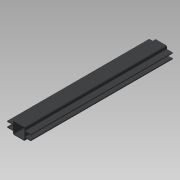
# Autodesk Inventor part: 9035
Saved by Autodesk Inventor 2013 (Build 170138000, 138)
## iProperties
Company: 80/20 Inc.
Created: 2014-04-23
Part Number: 9035
Material: Generic
Document SubType Name: Modeling
Density: 1 g/cm^3
Vendor: 80/20 Inc.
Engineer: Ross Bowman
Designer: Ross Bowman
Catalog Web Link: 8020.net
Material: 6105-T5 Aluminum
Author: Ross Bowman
Keywords: 80/20 , 8020 , T-Slot , Extrusion
Autodesk Inventor part; units mm, degrees
ref_plane "YZ Plane" through (0, 0, 0) normal (1, 0, 0) x (0, 1, 0)
ref_plane "XZ Plane" through (0, 0, 0) normal (0, 1, 0) x (-1, 0, 0)
ref_plane "XY Plane" through (0, 0, 0) normal (0, 0, 1) x (1, 0, 0)
sketch "Sketch1" plane through (0, 0, 0) normal (0, 0, 1) x (1, 0, 0)
  line L0 (-9.652, -11.176) -> (9.652, -11.176)
  arc A0 (-11.176, -9.652) -> (-9.652, -11.176) centre (-9.652, -9.652) ccw
  line L1 (-11.176, 9.652) -> (-11.176, -9.652)
  arc A1 (-9.652, 11.176) -> (-11.176, 9.652) centre (-9.652, 9.652) ccw
  line L2 (9.652, 11.176) -> (-9.652, 11.176)
  arc A2 (11.176, 9.652) -> (9.652, 11.176) centre (9.652, 9.652) ccw
  line L3 (11.176, -9.652) -> (11.176, 9.652)
  arc A3 (9.652, -11.176) -> (11.176, -9.652) centre (9.652, -9.652) ccw
  arc A4 (12.7, 6.731) -> (13.081, 6.35) centre (13.081, 6.731) ccw
  line L4 (12.7, 6.731) -> (12.7, 10.5918)
  arc A5 (12.7, 10.5918) -> (10.5918, 12.7) centre (10.5918, 10.5918) ccw
  line L5 (10.5918, 12.7) -> (-10.5918, 12.7)
  arc A6 (-10.5918, 12.7) -> (-12.7, 10.5918) centre (-10.5918, 10.5918) ccw
  line L6 (-12.7, 10.5918) -> (-12.7, 6.731)
  arc A7 (-13.081, 6.35) -> (-12.7, 6.731) centre (-13.081, 6.731) ccw
  line L7 (-13.081, 6.35) -> (-25.019, 6.35)
  arc A8 (-25.019, 6.35) -> (-25.4, 5.969) centre (-25.019, 5.969) ccw
  line L8 (-25.4, 5.969) -> (-25.4, 4.826)
  arc A9 (-25.4, 4.826) -> (-24.638, 4.064) centre (-24.638, 4.826) ccw
  line L9 (-24.638, 4.064) -> (-23.0632, 4.064)
  arc A10 (-23.0632, 4.064) -> (-22.6822, 4.445) centre (-23.0632, 4.445) ccw
  arc A11 (-22.3012, 4.826) -> (-22.6822, 4.445) centre (-22.3012, 4.445) ccw
  line L10 (-22.3012, 4.826) -> (-13.081, 4.826)
  arc A12 (-12.7, 4.445) -> (-13.081, 4.826) centre (-13.081, 4.445) ccw
  line L11 (-12.7, 4.445) -> (-12.7, -4.445)
  arc A13 (-13.081, -4.826) -> (-12.7, -4.445) centre (-13.081, -4.445) ccw
  line L12 (-13.081, -4.826) -> (-22.3012, -4.826)
  arc A14 (-22.6822, -4.445) -> (-22.3012, -4.826) centre (-22.3012, -4.445) ccw
  arc A15 (-22.6822, -4.445) -> (-23.0632, -4.064) centre (-23.0632, -4.445) ccw
  line L13 (-23.0632, -4.064) -> (-24.638, -4.064)
  arc A16 (-24.638, -4.064) -> (-25.4, -4.826) centre (-24.638, -4.826) ccw
  line L14 (-25.4, -4.826) -> (-25.4, -5.969)
  arc A17 (-25.4, -5.969) -> (-25.019, -6.35) centre (-25.019, -5.969) ccw
  line L15 (-25.019, -6.35) -> (-13.081, -6.35)
  arc A18 (-12.7, -6.731) -> (-13.081, -6.35) centre (-13.081, -6.731) ccw
  line L16 (-12.7, -6.731) -> (-12.7, -10.5918)
  arc A19 (-12.7, -10.5918) -> (-10.5918, -12.7) centre (-10.5918, -10.5918) ccw
  line L17 (-10.5918, -12.7) -> (10.5918, -12.7)
  arc A20 (10.5918, -12.7) -> (12.7, -10.5918) centre (10.5918, -10.5918) ccw
  line L18 (12.7, -10.5918) -> (12.7, -6.731)
  arc A21 (13.081, -6.35) -> (12.7, -6.731) centre (13.081, -6.731) ccw
  line L19 (13.081, -6.35) -> (25.019, -6.35)
  arc A22 (25.019, -6.35) -> (25.4, -5.969) centre (25.019, -5.969) ccw
  line L20 (25.4, -5.969) -> (25.4, -4.826)
  arc A23 (25.4, -4.826) -> (24.638, -4.064) centre (24.638, -4.826) ccw
  line L21 (24.638, -4.064) -> (23.0632, -4.064)
  arc A24 (23.0632, -4.064) -> (22.6822, -4.445) centre (23.0632, -4.445) ccw
  arc A25 (22.3012, -4.826) -> (22.6822, -4.445) centre (22.3012, -4.445) ccw
  line L22 (22.3012, -4.826) -> (13.081, -4.826)
  arc A26 (12.7, -4.445) -> (13.081, -4.826) centre (13.081, -4.445) ccw
  line L23 (12.7, -4.445) -> (12.7, 4.445)
  arc A27 (13.081, 4.826) -> (12.7, 4.445) centre (13.081, 4.445) ccw
  line L24 (13.081, 4.826) -> (22.3012, 4.826)
  arc A28 (22.6822, 4.445) -> (22.3012, 4.826) centre (22.3012, 4.445) ccw
  arc A29 (22.6822, 4.445) -> (23.0632, 4.064) centre (23.0632, 4.445) ccw
  line L25 (23.0632, 4.064) -> (24.638, 4.064)
  arc A30 (24.638, 4.064) -> (25.4, 4.826) centre (24.638, 4.826) ccw
  line L26 (25.4, 4.826) -> (25.4, 5.969)
  arc A31 (25.4, 5.969) -> (25.019, 6.35) centre (25.019, 5.969) ccw
  line L27 (25.019, 6.35) -> (13.081, 6.35)
  point P0 (0, 0)
  constraints: 64 point on circle, 56 end point, 32 centre point
extrude "Extrusion1" add sketch "Sketch1" against normal blind 304.8
body "Solid1"
